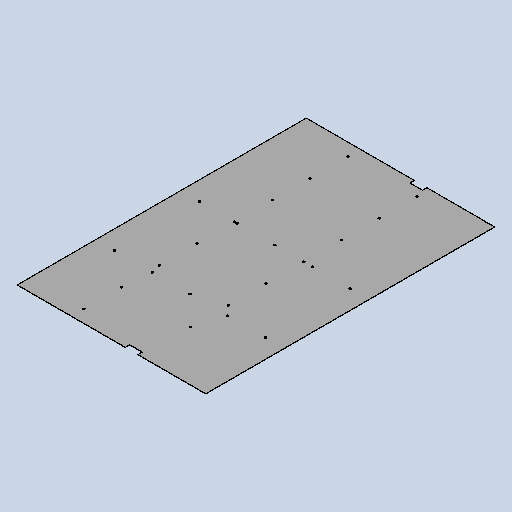
# Autodesk Inventor part: GnG R.3 floor sheet
Saved by Autodesk Inventor 2025.3 (Build 293356030, 356C)
## iProperties
Created: 2025-10-28
Part Number: GnG R.3 floor sheet
Material: Stainless Steel
Document SubType Name: Sheet Metal
Designer: admin
Mass: 82524.8 g
Surface Area: 69038.7 cm^2
Volume: 10315.6 cm^3
Density: 8 g/cm^3
Sheet Metal Rule: AISI304 3mm Die 32
Sheet Metal Width: 1500,000 mm
Sheet Metal Length: 2300,000 mm
Sheet Metal Area: 3450000,000 mm^2
Appearance: Default
Flat Pattern Width: 150 cm
Flat Pattern Length: 230 cm
Flat Pattern Area: 34500 cm^2
Stock Number: R 3
Author: admin
Autodesk Inventor part; units mm, degrees
ref_plane "YZ Plane" through (0, 0, 0) normal (1, 0, 0) x (0, 1, 0)
ref_plane "XZ Plane" through (0, 0, 0) normal (0, 1, 0) x (-1, 0, 0)
ref_plane "XY Plane" through (0, 0, 0) normal (0, 0, 1) x (1, 0, 0)
sketch "Sketch1" plane through (0, 0, 0) normal (0, 0, 1) x (1, 0, 0)
  line L0 (0, 0) -> (-1500, 0)
  line L1 (-1500, 0) -> (-1500, -2300)
  line L2 (-1500, -2300) -> (0, -2300)
  line L3 (0, -2300) -> (0, 0)
  line L4 (0, 0) -> (-40, 0)
  line L5 (-40, 0) -> (-40, -35)
  line L6 (-40, -35) -> (0, -35)
  line L7 (0, -35) -> (0, 0)
  line L8 (0, -2300) -> (-40, -2300)
  line L9 (-40, -2300) -> (-40, -2265)
  line L10 (-40, -2265) -> (0, -2265)
  line L11 (0, -2265) -> (0, -2300)
  line L12 (-1500, 0) -> (-1460, 0)
  line L13 (-1460, 0) -> (-1460, -35)
  line L14 (-1460, -35) -> (-1500, -35)
  line L15 (-1500, -35) -> (-1500, 0)
  line L16 (-1500, -2300) -> (-1460, -2300)
  line L17 (-1460, -2300) -> (-1460, -2265)
  line L18 (-1460, -2265) -> (-1500, -2265)
  line L19 (-1500, -2265) -> (-1500, -2300)
  line L20 (-640, -2300) -> (-540, -2300)
  line L21 (-540, -2300) -> (-540, -2265)
  line L22 (-540, -2265) -> (-640, -2265)
  line L23 (-640, -2265) -> (-640, -2300)
  line L24 (-640, 0) -> (-540, 0)
  line L25 (-540, 0) -> (-540, -35)
  line L26 (-540, -35) -> (-640, -35)
  line L27 (-640, -35) -> (-640, 0)
  point P0 (0, -35)
  point P1 (-40, 0)
  point P2 (-40, -2300)
  point P3 (0, -2265)
  point P4 (-540, -2300)
  point P5 (-540, 0)
  point P6 (-1460, 0)
  point P7 (-1500, -35)
  dimension "d22" = 1500
  dimension "d23" = 2300
  dimension "d24" = 40
  dimension "d25" = 35
  dimension "d28" = 100
  dimension "d29" = 500
  measures "d22" distance of L2.end L1.end
  measures "d23" distance of L1.end L0.end
  measures "d24" distance of L6.end L5.end
  measures "d25" distance of L5.end L4.end
  measures "d28" distance of L25.end L26.end
  measures "d29" distance between parallel lines of L5 L25
extrude "Plate1" add sketch "Sketch1" along normal blind 3 contours L3 L6 L5 L0 | L5 L6 L3 L10 L9 L2 L21 L22 L23 L17 L18 L1 L14 L13 L0 L27 L26 L25 | L3 L2 L9 L10 | L13 L14 L1 L0 | L18 L17 L2 L1
sketch "Sketch5" plane through (0, 0, 3) normal (0, 0, 1) x (1, 0, 0)
  line L0 (0, 0) -> (-540, 0) projected
  circle A0 centre (-54.849, 0) radius 2.5
  circle A1 centre (-69.3998, 0) radius 2.5
  line L1 (-77.6676, 0) -> (-82.6676, 0)
  line L2 (-82.6676, 0) -> (-82.6676, -2)
  line L3 (-82.6676, -2) -> (-77.6676, -2)
  line L4 (-77.6676, -2) -> (-77.6676, 0)
  line L5 (-89.1767, 0) -> (-94.1767, 0)
  line L6 (-94.1767, 0) -> (-94.1767, -2)
  line L7 (-94.1767, -2) -> (-89.1767, -2)
  line L8 (-89.1767, -2) -> (-89.1767, 0)
  line L9 (-100.2895, 0) -> (-105.2895, 0)
  line L10 (-105.2895, 0) -> (-105.2895, -2)
  line L11 (-105.2895, -2) -> (-100.2895, -2)
  line L12 (-100.2895, -2) -> (-100.2895, 0)
  dimension "d66" = 5
  dimension "d67" = 5
  dimension "d68" = 2
  constraints: 24 end point, 6 parallel, 6 point on line, 3 collinear, 3 horizontal, 3 perpendicular, 2 centre point, 1 equal radius
  measures "d66" diameter of A0
  measures "d67" distance of L3.end L2.end
  measures "d68" distance of L2.end L1.end
extrude "Cut1" cut sketch "Sketch5" against normal blind 3
sketch "Sketch6" plane through (0, 0, 3) normal (0, 0, 1) x (1, 0, 0)
  line L0 (-1500, -2300) -> (-1500, 0) construction
  line L1 (0, -2300) -> (-540, -2300) construction
  line L2 (0, 0) -> (0, -2300) construction
  line L3 (-540, 0) -> (-105.2895, 0) construction
  circle A0 centre (-520, -2200) radius 7.5
  line L4 (-540, -35) -> (-540, 0) construction
  line L5 (-640, -35) -> (-540, -35) construction
  line L6 (-640, 0) -> (-640, -35) construction
  line L7 (-1500, 0) -> (-640, 0) construction
  line L8 (-640, -2300) -> (-1500, -2300) construction
  line L9 (-640, -2265) -> (-640, -2300) construction
  line L10 (-540, -2265) -> (-640, -2265) construction
  line L11 (-540, -2300) -> (-540, -2265) construction
  line L12 (-520, -2300) -> (-520, 0) construction
  line L13 (-1070, 0) -> (-1070, -2300) construction
  line L14 (-1500, -1675) -> (0, -1675) construction
  line L15 (-1500, -1000) -> (0, -1000) construction
  circle A1 centre (-1070, -2200) radius 7.5
  circle A2 centre (-1350, -1675) radius 7.5
  circle A3 centre (-1350, -1000) radius 7.5
  circle A4 centre (-520, -1900) radius 7.5
  circle A5 centre (-1070, -1900) radius 7.5
  circle A6 centre (-520, -1600) radius 7.5
  circle A7 centre (-1070, -1600) radius 7.5
  circle A8 centre (-520, -1300) radius 7.5
  circle A9 centre (-1070, -1300) radius 7.5
  circle A10 centre (-520, -1000) radius 7.5
  circle A11 centre (-1070, -1000) radius 7.5
  circle A12 centre (-520, -700) radius 7.5
  circle A13 centre (-1070, -700) radius 7.5
  circle A14 centre (-520, -400) radius 7.5
  circle A15 centre (-1070, -400) radius 7.5
  circle A16 centre (-520, -100) radius 7.5
  circle A17 centre (-1070, -100) radius 7.5
  circle A18 centre (-520, 200) radius 7.5
  circle A19 centre (-1070, 200) radius 7.5
  circle A20 centre (-520, 500) radius 7.5
  circle A21 centre (-1070, 500) radius 7.5
  circle A22 centre (-520, 800) radius 7.5
  circle A23 centre (-1070, 800) radius 7.5
  circle A24 centre (-1050, -1675) radius 7.5
  circle A25 centre (-1050, -1000) radius 7.5
  circle A26 centre (-750, -1675) radius 7.5
  circle A27 centre (-750, -1000) radius 7.5
  circle A28 centre (-450, -1675) radius 7.5
  circle A29 centre (-450, -1000) radius 7.5
  circle A30 centre (-150, -1675) radius 7.5
  circle A31 centre (-150, -1000) radius 7.5
  circle A32 centre (150, -1675) radius 7.5
  circle A33 centre (150, -1000) radius 7.5
  circle A34 centre (450, -1675) radius 7.5
  circle A35 centre (450, -1000) radius 7.5
  arc A36 (-57.349, 0) -> (-52.349, 0) centre (-54.849, 0) ccw projected
  line L16 (-66.8998, 0) -> (-57.349, 0) projected
  arc A37 (-71.8998, 0) -> (-66.8998, 0) centre (-69.3998, 0) ccw projected
  line L17 (-77.6676, 0) -> (-71.8998, 0) projected
  line L18 (-77.6676, 0) -> (-77.6676, -2) projected
  line L19 (-77.6676, -2) -> (-82.6676, -2) projected
  line L20 (-82.6676, -2) -> (-82.6676, 0) projected
  line L21 (-89.1767, 0) -> (-82.6676, 0) projected
  line L22 (-89.1767, 0) -> (-89.1767, -2) projected
  line L23 (-89.1767, -2) -> (-94.1767, -2) projected
  line L24 (-94.1767, -2) -> (-94.1767, 0) projected
  line L25 (-100.2895, 0) -> (-94.1767, 0) projected
  line L26 (-100.2895, 0) -> (-100.2895, -2) projected
  line L27 (-100.2895, -2) -> (-105.2895, -2) projected
  line L28 (-105.2895, -2) -> (-105.2895, 0) projected
  line L29 (-52.349, 0) -> (0, 0) projected
  dimension "d41" = 15
  dimension "d46" = 520
  dimension "d47" = 1070
  dimension "d48" = 625
  dimension "d49" = 1300
  dimension "d50" = 100
  dimension "d51" = 150
  dimension "d54" = 300
  dimension "d61" = 300
  constraints: 36 centre point, 9 point on line, 8 end point, 3 equal radius, 3 perpendicular, 2 midpoint, 1 horizontal, 1 horizontal alignment, 1 vertical, 1 vertical alignment, 64 other
  measures "d41" diameter of A0
  measures "d46" distance between parallel lines of L12 L2
  measures "d47" distance between parallel lines of L13 L2
  measures "d48" distance between parallel lines of L8 L14
  measures "d49" distance between parallel lines of L15 L8
  measures "d50" distance from line of L1 A0.centre
  measures "d51" distance from line of L0 A2.centre
  measures "d54" distance of A0.centre A4.centre
  measures "d61" distance of A2.centre A24.centre
extrude "Cut2" cut sketch "Sketch6" against normal blind 3 contours A1 | A2 | A3 | A4 | A5 | A6 | A7 | A8 | A9 | A10 | A11 | A12 | A13 | A14 | A15 | A16 | A17 | A18 | A19 | A20 | A21 | A22 | A23 | A24 | A25 | A26 | A27 | A28 | A29 | A30 | A31 | A32 | A33 | A34 | A35
equation "\"d39\" = Thickness"
equation "\"d61\" = d54"
equation "\"d44\" = Thickness"
equation "\"d2\" = Thickness"
equation "\"BendReliefWidth\" = Thickness"
equation "\"BendReliefDepth\" = 0.5 * Thickness"
equation "\"CornerReliefSize\" = 4 * Thickness"
equation "\"MinimumRemnant\" = 2 * Thickness"
equation "\"TransitionRadius\" = BendRadius"
equation "\"JacobiRadiusSize\" = BendRadius"
equation "\"GapSize\" = Thickness"
equation "\"Thickness\" = 3"
equation "\"BendRadius\" = 5"
body "Solid1"
